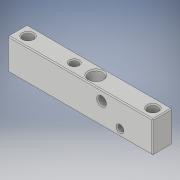
# Autodesk Inventor part: holes1
Saved by Autodesk Inventor 2017 (Build 210142000, 142)
## iProperties
Created: 2017-04-13
Part Number: holes1
Material: Generic
Document SubType Name: Modeling
Designer: 167942
Density: 1 g/cm^3
Appearance: Default
Author: 167942
Autodesk Inventor part; units mm, degrees
ref_plane "YZ Plane" through (0, 0, 0) normal (1, 0, 0) x (0, 1, 0)
ref_plane "XZ Plane" through (0, 0, 0) normal (0, 1, 0) x (-1, 0, 0)
ref_plane "XY Plane" through (0, 0, 0) normal (0, 0, 1) x (1, 0, 0)
sketch "Sketch1" plane through (0, 0, 0) normal (1, 0, 0) x (0, 1, 0)
  line L0 (0, 0) -> (25.4, 0)
  line L1 (25.4, 0) -> (25.4, -15.875)
  line L2 (25.4, -15.875) -> (0, -15.875)
  line L3 (0, -15.875) -> (0, 0)
  dimension "d0" = 25.4
  dimension "d1" = 15.875
  constraints: 8 end point, 2 parallel, 1 horizontal, 1 perpendicular
  measures "d0" distance of L1.end L2.end
  measures "d1" distance of L2.end L0.start
extrude "Extrusion1" add sketch "Sketch1" along normal blind 117.475
chamfer "Chamfer1" distance 0.762 angle 45 11 edges at (117.475, 12.7, 0) (117.475, 12.7, -15.875) (117.475, 0, -7.9375) (58.7375, 0, 0) (58.7375, 25.4, 0) (58.7375, 25.4, -15.875) (0, 12.7, 0) (0, 25.4, -7.9375) (0, 12.7, -15.875) (0, 0, -7.9375) (58.7375, 0, -15.875)
sketch "Sketch2" plane through (0.762, 25.4, -15.113) normal (0, 1, 0) x (1, 0, 0)
  line L0 (0, -15.113) -> (115.951, -15.113) projected
  line L1 (0, -15.113) -> (7.9375, -15.113)
  line L2 (7.9375, -15.113) -> (7.9375, -7.1755)
  point P0 (-0.762, -15.113)
  dimension "d7" = 7.9375
  dimension "d8" = 7.9375
  constraints: 4 end point, 1 perpendicular, 1 point on line
  measures "d7" distance of L0.start L1.end
  measures "d8" distance of L1.end L2.end
hole "Hole1" at (8.6995, 25.4, -7.9375) direction (0, -1, 0) diameter 7.9375 end through all countersink diameter 9.525 countersink angle 82
sketch "Sketch3" plane through (0.762, 25.4, -15.113) normal (0, 1, 0) x (1, 0, 0)
  line L0 (116.713, 0) -> (116.713, -14.351) projected
  line L1 (116.713, -7.1755) -> (45.2755, -7.1755)
  point P0 (-0.762, -15.113)
  dimension "d16" = 71.4375
  constraints: 2 end point, 1 horizontal, 1 midpoint
  measures "d16" distance of L1.start L1.end
hole "Hole2" at (46.0375, 25.4, -7.9375) direction (0, -1, 0) diameter 6.35 end through all countersink diameter 7.9375 countersink angle 82
sketch "Sketch4" plane through (0.762, 25.4, -15.113) normal (0, 1, 0) x (1, 0, 0)
  line L0 (116.713, 0) -> (116.713, -14.351) projected
  line L1 (116.713, -7.1755) -> (62.738, -7.1755)
  point P0 (-0.762, -15.113)
  dimension "d24" = 53.975
  constraints: 2 end point, 1 horizontal, 1 midpoint
  measures "d24" distance of L1.start L1.end
hole "Hole3" at (63.5, 25.4, -7.9375) direction (0, -1, 0) diameter 11.1125 end through all countersink diameter 12.7 countersink angle 82
sketch "Sketch5" plane through (0.762, 25.4, -15.113) normal (0, 1, 0) x (1, 0, 0)
  line L0 (116.713, 0) -> (116.713, -14.351) projected
  line L1 (116.713, -7.1755) -> (108.7755, -7.1755)
  point P0 (-0.762, -15.113)
  dimension "d32" = 7.9375
  constraints: 2 end point, 1 horizontal, 1 midpoint
  measures "d32" distance of L1.start L1.end
hole "Hole4" at (109.5375, 25.4, -7.9375) direction (0, -1, 0) diameter 7.9375 end through all countersink diameter 9.525 countersink angle 82
sketch "Sketch6" plane through (0.762, 0.762, 0) normal (0, 0, 1) x (1, 0, 0)
  line L0 (111.9534, -0.762) -> (111.9534, 4.8006) construction
  line L1 (117.1134, 4.8006) -> (90.1259, 4.8006) construction
  point P0 (-0.762, -0.762)
  dimension "d40" = 5.5626
  dimension "d41" = 26.9875
  constraints: 4 end point, 1 horizontal, 1 vertical
  measures "d40" distance of L0.start L0.end
  measures "d41" distance of L1.start L1.end
hole "Hole5" at (90.8879, 5.5626, 0) direction (0, 0, -1) diameter 4.7625 end through all countersink diameter 6.35 countersink angle 82
sketch "Sketch7" plane through (0.762, 0.762, 0) normal (0, 0, 1) x (1, 0, 0)
  line L0 (114.57, -0.762) -> (114.57, 16.7005)
  line L1 (116.5466, 16.7005) -> (75.2716, 16.7005)
  point P0 (-0.762, -0.762)
  dimension "d49" = 17.4625
  dimension "d50" = 41.275
  constraints: 4 end point, 1 horizontal, 1 vertical
  measures "d49" distance of L0.start L0.end
  measures "d50" distance of L1.start L1.end
hole "Hole6" at (76.0336, 17.4625, 0) direction (0, 0, -1) diameter 6.35 end through all countersink diameter 7.9375 countersink angle 82
chamfer "Chamfer2" distance 0.762 angle 45 1 edges at (117.475, 25.4, -7.9375)
body "Solid1"
